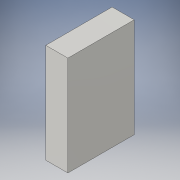
# Autodesk Inventor part: Pool Controller
Saved by Autodesk Inventor 2016 (Build 200138000, 138)
## iProperties
Created: 2015-05-30
Part Number: Pool Controller
Material: Aluminum 6061
Document SubType Name: Modeling
Designer: steele
Density: 2.7 g/cm^3
Appearance: White
Author: steele
Autodesk Inventor part; units mm, degrees
ref_plane "YZ Plane" through (0, 0, 0) normal (1, 0, 0) x (0, 1, 0)
ref_plane "XZ Plane" through (0, 0, 0) normal (0, 1, 0) x (-1, 0, 0)
ref_plane "XY Plane" through (0, 0, 0) normal (0, 0, 1) x (1, 0, 0)
sketch "Sketch1" plane through (0, 0, 0) normal (1, 0, 0) x (0, 1, 0)
  line L0 (-228.6, 152.4) -> (-228.6, -152.4)
  line L1 (-228.6, -152.4) -> (228.6, -152.4)
  line L2 (228.6, -152.4) -> (228.6, 152.4)
  line L3 (228.6, 152.4) -> (-228.6, 152.4)
  line L4 (-228.6, 152.4) -> (228.6, -152.4) construction
  line L5 (-228.6, -152.4) -> (228.6, 152.4) construction
  point P0 (0, 0)
  dimension "d0" = 457.2
  dimension "d1" = 304.8
  constraints: 12 end point, 2 midpoint, 2 parallel, 1 perpendicular, 1 vertical
  measures "d0" distance of L2.end L0.start
  measures "d1" distance of L1.end L2.end
extrude "Extrusion1" add sketch "Sketch1" along normal mid plane 101.6
body "Solid1"
